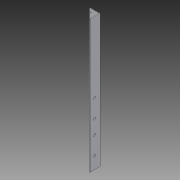
# Autodesk Inventor part: 26in Angle Channel CIM Mount Left
Saved by Autodesk Inventor 2013 (Build 170138000, 138)
## iProperties
Created: 2013-01-27
Part Number: 26in Angle Channel CIM Mount Left
Material: Aluminum 6061
Document SubType Name: Modeling
Designer: Naphat
Density: 1 g/cm^3
Author: Naphat
Autodesk Inventor part; units mm, degrees
ref_plane "YZ Plane" through (0, 0, 0) normal (1, 0, 0) x (0, 1, 0)
ref_plane "XZ Plane" through (0, 0, 0) normal (0, 1, 0) x (-1, 0, 0)
ref_plane "XY Plane" through (0, 0, 0) normal (0, 0, 1) x (1, 0, 0)
sketch "Sketch1" plane through (0, 0, 0) normal (0, 1, 0) x (-1, 0, 0)
  line L0 (0, 0) -> (50, 0)
  line L1 (50, 0) -> (50, 3)
  line L2 (0, 0) -> (0, 50)
  line L3 (0, 50) -> (3, 50)
  line L4 (3, 50) -> (3, 3)
  line L5 (3, 3) -> (50, 3)
  dimension "d0" = 50
  dimension "d1" = 3
  dimension "d2" = 50
  dimension "d3" = 3
  constraints: 12 end point, 3 perpendicular, 2 parallel, 1 horizontal
  measures "d0" distance of L0.start L0.end
  measures "d1" distance of L0.end L1.end
  measures "d2" distance of L0.start L2.end
  measures "d3" distance of L2.end L3.end
extrude "Extrusion1" add sketch "Sketch1" along normal blind 660.4
sketch "Sketch5" plane through (-3, 0, 3) normal (-1, 0, 0) x (0, 0, 1)
  circle A0 centre (24.5, 59.2629) radius 4.8387
  circle A1 centre (24.5, 149.2629) radius 4.8387
  circle A2 centre (24.5, 219.0371) radius 4.8387
  circle A3 centre (24.5, 309.0371) radius 4.8387
  line L0 (0, 0) -> (47, 0) projected
  line L1 (0, 0) -> (0, 660.4) projected
  line L2 (-136.6387, 184.15) -> (192.6114, 184.15) construction
  line L3 (47, 0) -> (47, 660.4) projected
  line L4 (-3, 0) -> (-3, 660.4) construction
  dimension "d68" = 90
  dimension "d70" = 90
  dimension "d71" = 69.7742
  dimension "d72" = 184.15
  dimension "d73" = 34.8871
  dimension "d74" = 34.8871
  dimension "d78" = 59.2629
  dimension "d79" = 50
  dimension "d102" = 22.5
  constraints: 4 centre point, 2 end point, 2 vertical alignment, 1 perpendicular
  measures "d68" distance of A2.centre A3.centre
  measures "d70" distance of A0.centre A1.centre
  measures "d71" distance of A1.centre A2.centre
  measures "d72" distance between parallel lines of L0 L2
  measures "d73" distance from line of A1.centre L2
  measures "d74" distance from line of A2.centre L2
  measures "d78" distance from line of A0.centre L0
  measures "d79" distance between parallel lines of L3 L4
  measures "d102" distance from line of L3 A3.centre
sketch "Sketch6" plane through (-50, 0, 3) normal (0, 0, 1) x (1, 0, 0)
  line L0 (0, 0) -> (47, 0) projected
  line L1 (47, 0) -> (47, 660.4) projected
  line L2 (0, 660.4) -> (47, 660.4) projected
  line L3 (0, 0) -> (0, 660.4) projected
  line L4 (0, 0) -> (47, 0) projected
  line L5 (47, 0) -> (47, 660.4) projected
  line L6 (0, 660.4) -> (47, 660.4) projected
  line L7 (0, 0) -> (0, 660.4) projected
  line L8 (50, 0) -> (50, 660.4) projected
  line L9 (47, 660.4) -> (50, 660.4) projected
  line L10 (0, 644.4) -> (50, 644.4) construction
  circle A0 centre (6.35, 644.4) radius 3.175
  circle A1 centre (40.65, 644.4) radius 3.175
  line L11 (50, 16) -> (0, 16) construction
  circle A2 centre (40.65, 16) radius 3.175
  circle A3 centre (6.35, 16) radius 3.175
  dimension "d80" = 16
  dimension "d81" = 6.35
  dimension "d82" = 6.35
  dimension "d83" = 6.35
  dimension "d84" = 6.35
  dimension "d85" = 16
  dimension "d86" = 6.35
  dimension "d87" = 6.35
  constraints: 8 point on line, 4 centre point, 4 end point, 2 vertical alignment, 1 parallel, 1 perpendicular
  measures "d80" distance between parallel lines of L2 L10
  measures "d81" diameter of A0
  measures "d82" diameter of A1
  measures "d83" distance from line of A1.centre L1
  measures "d84" distance from line of L3 A0.centre
  measures "d85" distance between parallel lines of L0 L11
  measures "d86" diameter of A2
  measures "d87" diameter of A3
hole "Hole1" at (-9.35, 644.4, 3) at (-43.65, 644.4, 3) at (-9.35, 16, 3) at (-43.65, 16, 3) direction (0, 0, -1) diameter 6.35 depth 3 tip angle 118
hole "Hole2" at (-3, 59.2629, 27.5) at (-3, 149.2629, 27.5) at (-3, 219.0371, 27.5) at (-3, 309.0371, 27.5) direction (1, 0, 0) diameter 12 depth 3 tip angle 118
equation "\"d68\" = d70"
equation "\"d73\" = 0.5 * d71"
equation "\"d74\" = 0.5 * d71"
body "Solid1"
